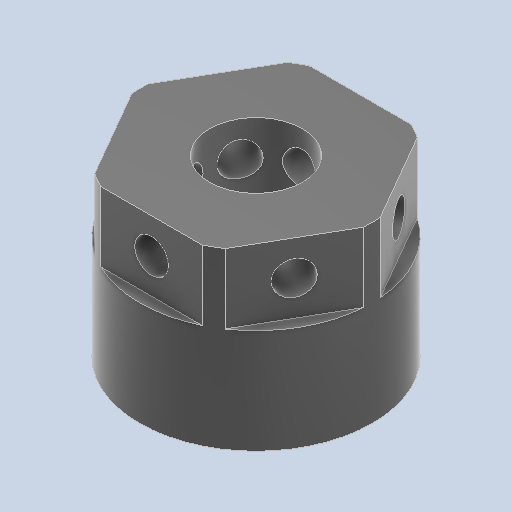
# Autodesk Inventor part: comutator_plastic
Saved by Autodesk Inventor 2025 (Build 290162000, 162)
## iProperties
Created: 2026-08-07
Part Number: comutator_plastic
Material: Ogólny
Document SubType Name: Modeling
Designer: zzapa
Density: 1 g/cm^3
Appearance: Gładki — czarny
Author: zzapa
Autodesk Inventor part; units mm, degrees
ref_plane "YZ Plane" through (0, 0, 0) normal (1, 0, 0) x (0, 1, 0)
ref_plane "XZ Plane" through (0, 0, 0) normal (0, 1, 0) x (-1, 0, 0)
ref_plane "XY Plane" through (0, 0, 0) normal (0, 0, 1) x (1, 0, 0)
sketch "Szkic1" plane through (0, 0, 0) normal (0, 1, 0) x (-1, 0, 0)
  circle A0 centre (0, 0) radius 10
  circle A1 centre (0, 0) radius 4
  dimension "d0" = 20
  dimension "d1" = 8
  constraints: 2 centre point, 2 coincident
  measures "d0" diameter of A0
  measures "d1" diameter of A1
extrude "Wyciągnięcie proste1" add sketch "Szkic1" along normal blind 15
sketch "Szkic2" plane through (0, 0, 0) normal (1, 0, 0) x (0, 1, 0)
  line L0 (15, -10) -> (15, 10) projected
  line L1 (0, -10) -> (0, 10) projected
  line L2 (15, -4) -> (0, -4) projected
  line L3 (0, -10) -> (15, -10) projected
  line L4 (15, -10) -> (9, -10)
  line L5 (9, -10) -> (9, -9)
  line L6 (9, -9) -> (15, -9)
  line L7 (15, -9) -> (15, -10)
  point P0 (0, 0)
  point P1 (9, -10)
  dimension "d9" = 1
  dimension "d10" = 6
  constraints: 8 end point, 2 collinear, 2 parallel, 1 horizontal, 1 perpendicular
  measures "d9" distance of L4.end L5.end
  measures "d10" distance of L5.end L6.end
extrude "Wyciągnięcie proste2" cut sketch "Szkic2" along normal through all both and the other way through all contours L3 L5 L6 L0
pattern_circular "Szyk kołowy1" count 6 over 360 about axis through (0, -10, 0) along (0, 1, 0) of "Wyciągnięcie proste2"
sketch "Szkic3" plane through (4.3589, 15, -9) normal (0, 0, -1) x (-1, 0, 0)
  line L0 (8.7178, 0) -> (8.7178, -6) projected
  line L1 (0, 0) -> (8.7178, 0) projected
  line L2 (0, -6) -> (0, 0) projected
  line L3 (0, -6) -> (8.7178, -6) projected
  line L4 (0, 0) -> (8.7178, 0) projected
  line L5 (0, -6) -> (8.7178, -6) projected
  line L6 (4.3589, -6) -> (4.3589, 0)
  point P0 (4.3589, -15)
  point P1 (4.3589, -3)
  dimension "d21" = 3
  constraints: 3 midpoint, 2 end point
  measures "d21" distance from line of L1 point (4.359, -3)
hole "Otwór1" at (0, 12, -9) direction (0, 0, 1) diameter 2.9 depth 9
pattern_circular "Szyk kołowy2" count 6 over 360 about axis through (0, -10, 0) along (0, 1, 0) of "Otwór1"
equation "\"d0\" = commutator_plastic_D"
equation "\"d1\" = commutator_plastic_shaft_d"
equation "\"d2\" = commutator_plastic_h"
equation "\"d9\" = commutator_plastic_insert_cut_deepness"
equation "\"d10\" = commutator_plastic_insert_cut_length"
equation "\"d21\" = commutator_plastic_insert_pos"
equation "\"d11\" = insert_m2_d"
equation "\"insert_m2_d\" = 2.9"
equation "\"insert_m2_h\" = 7"
equation "\"insert_m2_corner\" = 0.5"
equation "\"insert_m2_pocket_d\" = 2.6"
equation "\"insert_m2_pocket_D\" = 4.5"
equation "\"insert_m2_pocket_nut_h\" = 1.5"
equation "\"stator_out_d\" = 2.5"
equation "\"stator_h\" = 45"
equation "\"mag_size_x\" = 7"
equation "\"mag_size_y\" = 3"
equation "\"mag_corner_r\" = 0.4"
equation "\"magnet_ring_r\" = 27.5"
equation "\"magnet_ring_d\" = 3.3"
equation "\"magnet_ring_h\" = 36"
equation "\"magnet_ring_pocket_mag_size_x\" = 7.1"
equation "\"magnet_ring_pocket_mag_size_y\" = 3.1"
equation "\"magnet_ring_pocket_mag_size_z\" = 10.3"
equation "\"magnet_ring_pocket_radial_cut\" = 1.4"
equation "\"casing_d\" = 3"
equation "\"rotor_out_r\" = 23"
equation "\"rotor_coil_groove_in_r\" = 17"
equation "\"rotor_coil_groove_ang\" = 18deg"
equation "\"rotor_core_r\" = 15"
equation "\"rotor_coil_groove_in_correction_r\" = 18"
equation "\"rotor_plastic_h\" = 32"
equation "\"rotor_teeth_d\" = 1.5"
equation "\"rotor_plastic_insert_r\" = 37"
equation "\"shaft_d\" = 8"
equation "\"shaft_lock_1_d\" = 8"
equation "\"shaft_lock_1_D\" = 44"
equation "\"shaft_lock_1_h1\" = 3.5"
equation "\"shaft_lock_1_corner\" = 2"
equation "\"shaft_lock_1_rotor_insert_grove_d_in\" = 36"
equation "\"shaft_lock_1_rotor_insert_grove_width_out\" = 5.5"
equation "\"shaft_lock_1_rotor_insert_grove_width_in\" = 7.6"
equation "\"shaft_lock_1_rotor_insert_r\" = 37"
equation "\"shaft_lock_1_shaft_insert_axial_cut_out_width\" = 12"
equation "\"shaft_lock_1_shaft_insert_axial_cut_in_width\" = 5.4"
equation "\"shaft_lock_1_shaft_insert_pos\" = 2.5"
equation "\"shaft_lock_1_shaft_insert_corner\" = 2"
equation "\"shaft_lock_1_shaft_insert_corner_finish\" = 0.5"
equation "\"shaft_lock_2_d\" = 8"
equation "\"shaft_lock_2_D\" = 44"
equation "\"shaft_lock_2_h1\" = 3.5"
equation "\"shaft_lock_2_corner\" = 2"
equation "\"shaft_lock_2_rotor_insert_grove_d_in\" = 36"
equation "\"shaft_lock_2_rotor_insert_grove_width_out\" = 5.5"
equation "\"shaft_lock_2_rotor_insert_grove_width_in\" = 7.6"
equation "\"shaft_lock_2_rotor_insert_r\" = 37"
equation "\"shaft_lock_2_shaft_insert_axial_cut_out_width\" = 12"
equation "\"shaft_lock_2_shaft_insert_axial_cut_in_width\" = 5.4"
equation "\"shaft_lock_2_shaft_insert_pos\" = 2.5"
equation "\"shaft_lock_2_shaft_insert_corner\" = 2"
equation "\"shaft_lock_2_shaft_insert_corner_finish\" = 0.5"
equation "\"commutator_plastic_D\" = 20"
equation "\"commutator_plastic_h\" = 15"
equation "\"commutator_plate_D\" = 22"
equation "\"commutator_plate_d\" = 1"
equation "\"commutator_plate_ang\" = 55deg"
equation "\"commutator_plate_h\" = 15"
equation "\"commutator_plastic_shaft_d\" = 8"
equation "\"commutator_plastic_insert_cut_deepness\" = 1"
equation "\"commutator_plastic_insert_cut_length\" = 6"
equation "\"commutator_plastic_insert_pos\" = 3"
equation "\"commutator_plate_insert_pos\" = 3"
equation "\"casing_lock_hole_r\" = 14"
equation "\"casing_lock_h\" = 8"
equation "\"casing_stator_fix_r\" = 23"
equation "\"casing_stator_fix_h\" = 6"
equation "\"magnet_ring_insert_part_lengthen\" = 8"
equation "\"casing_sidebar_length\" = 3"
equation "\"casing_vent_hole_length\" = 4"
equation "\"casing_vent_hole_width\" = 7"
equation "\"sleeve_cup_r\" = 22"
equation "\"sleeve_cup_h\" = 3"
equation "\"sleeve_d\" = 3"
equation "\"sleeve_in_r\" = 11"
equation "\"casing_head_insert_r\" = 19"
equation "\"sleeve_head_insert_r\" = 19"
equation "\"magnet_ring_insert_part_radius_cut\" = 0.17"
equation "\"magnet_ring_insert_part_axial_flat_cut\" = 0.17"
equation "\"magnet_ring_insert_pos\" = 4"
equation "\"casing_radial_stator_insert_pos\" = 18.1"
equation "\"stator_radial_screw_d\" = 4"
equation "\"stator_radial_screw_pos\" = 4"
equation "\"rotor_sleeve_out_D\" = 10.5"
equation "\"rotor_sleeve_in_D\" = 8"
equation "\"rotor_sleeve_h\" = 32"
equation "\"carbon_brush_batt_d\" = 5"
